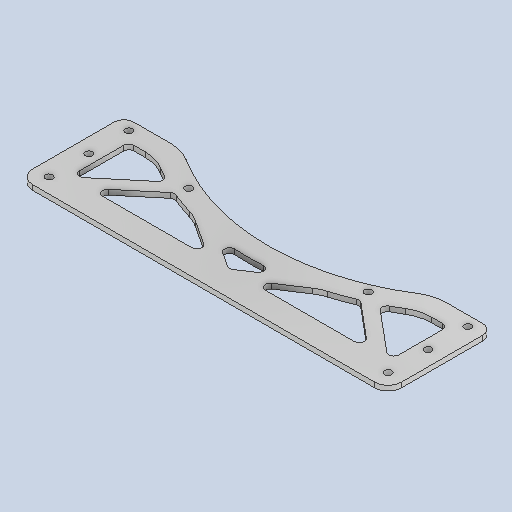
# Autodesk Inventor part: Custom Aluminum Intake
Saved by Autodesk Inventor 2025.1 (Build 291241020, 241B)
## iProperties
Created: 2024-12-30
Part Number: Custom Aluminum Intake
Material: Generic
Document SubType Name: Modeling
Designer: Juan
Density: 1 g/cm^3
Appearance: Default
Author: Juan
Autodesk Inventor part; units mm, degrees
ref_plane "YZ Plane" through (0, 0, 0) normal (1, 0, 0) x (0, 1, 0)
ref_plane "XZ Plane" through (0, 0, 0) normal (0, 1, 0) x (-1, 0, 0)
ref_plane "XY Plane" through (0, 0, 0) normal (0, 0, 1) x (1, 0, 0)
sketch "Sketch1" plane through (0, 0, 0) normal (0, 1, 0) x (-1, 0, 0)
  line L0 (0, 0) -> (-228.6, 0)
  line L1 (-228.6, 0) -> (-228.6, -82.55)
  line L2 (0, 0) -> (0, -82.55)
  line L3 (-228.6, 0) -> (-222.25, 0)
  circle A0 centre (-222.25, -6.35) radius 2.3241
  circle A1 centre (-222.25, -31.75) radius 2.3241
  line L4 (-228.6, 0) -> (-114.3, 0)
  line L5 (-114.3, 0) -> (-114.3, 9.4502)
  circle A2 centre (-222.25, -69.85) radius 2.3241
  circle A3 centre (-6.35, -6.35) radius 2.3241
  circle A4 centre (-6.35, -31.75) radius 2.3241
  circle A5 centre (-6.35, -69.85) radius 2.3241
  line L6 (-228.6, -82.55) -> (-215.9, -82.55)
  line L7 (0, -82.55) -> (-12.7, -82.55)
  line L8 (-114.3, 0) -> (-114.3, -38.1)
  arc A6 (-12.7, -82.55) -> (-215.9, -82.55) centre (-114.3, -176.4393) ccw
  line L9 (-228.6, 0) -> (-231.775, 0)
  line L10 (-231.775, 0) -> (-231.775, -82.55)
  line L11 (-231.775, -82.55) -> (-228.6, -82.55)
  line L12 (-228.6, 0) -> (-228.6, 3.175)
  line L13 (-228.6, 3.175) -> (-231.775, 3.175)
  line L14 (-231.775, 3.175) -> (-231.775, 0)
  line L15 (-228.6, 3.175) -> (0, 3.175)
  line L16 (0, 3.175) -> (0, 0)
  line L17 (0, 0) -> (3.175, 0)
  line L18 (3.175, 0) -> (3.175, 3.175)
  line L19 (3.175, 3.175) -> (0, 3.175)
  line L20 (3.175, 0) -> (3.175, -82.55)
  line L21 (3.175, -82.55) -> (0, -82.55)
  line L22 (-222.25, -69.85) -> (-222.25, -57.15)
  circle A7 centre (-222.25, -57.15) radius 2.3241
  line L23 (-6.35, -69.85) -> (-6.35, -57.15)
  circle A8 centre (-6.35, -57.15) radius 2.3241
  line L24 (-228.6, -63.5) -> (-194.1904, -63.5)
  line L25 (3.175, -63.5) -> (-34.4096, -63.5)
  line L26 (-231.775, -63.5) -> (-194.1904, -63.5)
  line L27 (-228.6, -69.85) -> (-221.3121, -69.85)
  arc A9 (-7.2879, -69.85) -> (-221.3121, -69.85) centre (-114.3, -176.4393) ccw
  line L28 (-7.2879, -69.85) -> (0, -69.85)
  line L29 (-228.6, -12.7) -> (0, -12.7)
  line L30 (-12.7, 0) -> (-12.7, -82.55)
  line L31 (-215.9, 0) -> (-215.9, -82.55)
  line L32 (-12.7, -12.7) -> (-46.8946, -41.275)
  line L33 (-12.7, -12.7) -> (-25.4, -12.7)
  line L34 (-25.4, -12.7) -> (-55.0732, -37.4966)
  line L35 (-114.3, -12.7) -> (-92.459, -26.9875)
  line L36 (-114.3, -12.7) -> (-101.6, -12.7)
  line L37 (-101.6, -12.7) -> (-73.6787, -30.965)
  line L38 (-215.9, -12.7) -> (-181.7054, -41.275)
  line L39 (-203.2, -12.7) -> (-173.5268, -37.4966)
  line L40 (-114.3, -12.7) -> (-136.141, -26.9875)
  line L41 (-127, -12.7) -> (-154.9213, -30.965)
  point P0 (-225.425, 0)
  point P1 (-215.9, -12.7)
  point P2 (-215.9, -63.5)
  point P3 (-214.5875, -63.5)
  point P4 (-14.0125, -63.5)
  point P5 (-12.7, -63.5)
  dimension "d0" = 228.6
  dimension "d1" = 82.55
  dimension "d2" = 6.35
  dimension "d4" = 4.6482
  dimension "d6" = 4.6482
  dimension "d7" = 114.3
  dimension "d9" = 4.6482
  dimension "d10" = 6.35
  dimension "d11" = 31.75
  dimension "d12" = 69.85
  dimension "d14" = 12.7
  dimension "d15" = 12.7
  dimension "d16" = 38.1
  dimension "d20" = 3.175
  dimension "d21" = 3.175
  dimension "d22" = 3.175
  dimension "d27" = 12.7
  dimension "d28" = 4.6482
  dimension "d29" = 12.7
  dimension "d30" = 4.6482
  dimension "d35" = 12.7
  dimension "d36" = 15.875
  dimension "d37" = 12.7
  dimension "d38" = 12.7
  dimension "d39" = 12.7
  dimension "d40" = 12.7
  constraints: 84 end point, 13 point on line, 11 point on circle, 10 centre point, 10 symmetric about line, 9 perpendicular, 6 parallel, 6 vertical, 4 horizontal, 3 midpoint, 2 coincident, 2 collinear, 5 other
  measures "d0" distance of L0.start L0.end
  measures "d1" distance of L0.end L1.end
  measures "d2" distance of L0.end L3.end
  measures "d4" diameter of A0
  measures "d6" diameter of A1
  measures "d7" distance of L0.end L4.end
  measures "d9" diameter of A2
  measures "d10" distance from line of A0.centre L0
  measures "d11" distance from line of L0 A1.centre
  measures "d12" vertical distance of point (-225.425, 0) L22.start
  measures "d14" distance of L1.end L6.end
  measures "d15" distance of L2.end L7.end
  measures "d16" distance of L4.end L8.end
  measures "d20" distance of L0.end L9.end
  measures "d21" distance of L0.end L12.end
  measures "d22" distance of L0.start L17.end
  measures "d27" distance of L22.start L22.end
  measures "d28" diameter of A7
  measures "d29" distance of L23.start L23.end
  measures "d30" diameter of A8
  measures "d35" radial gap between concentric circles of A6 A9
  measures "d36" distance between parallel lines of L15 L29
  measures "d37" distance between parallel lines of L2 L30
  measures "d38" distance between parallel lines of L1 L31
  measures "d39" distance of L32.start L33.end
  measures "d40" distance of L35.start L36.end
extrude "Extrusion1" add sketch "Sketch1" against normal blind 3.175 contours L2 L29 L30 L0 | L30 L29 L8 L0 | L2 L25 L30 L29 | L8 L29 L31 L0 | L32 A9 L34 L29 | L30 L25 A9 L32 | L2 L28 A5 L23 L25 | L31 L29 L1 L0 | L35 A9 L8 | L40 A9 L41 L29 | L29 L37 A9 L35 | L8 A9 L40 | L34 A9 L37 L29 | L30 A9 L25 | L25 L23 A5 A9 L30 | A9 L25 A6 L8 | L2 L7 L30 A9 A5 L28 | L31 L24 L1 L29 | L38 A9 L24 L31 | L29 L39 A9 L38 | L8 A6 L24 A9 | L41 A9 L39 L29 | A9 L30 A6 L25 | L31 A9 A2 L22 L24 | L24 A9 L31 | L24 L22 A2 L27 L1 | L24 A6 L31 A9 | L31 L6 L1 L27 A2 A9 | A7 | A8
fillet "Fillet1" radius 8.4667 4 edges at (228.6, -1.5875, -82.55) (215.9, -1.5875, -82.55) (12.7, -1.5875, -82.55) (0, -1.5875, -82.55)
extrude "Extrusion2" add sketch "Sketch1" against normal blind 3.175 contours L2 L29 L30 L0 | L17 L20 L25 L2 | L0 L5 L15 L16 | L16 L19 L18 L17 | L30 L29 L8 L0 | L2 L25 L30 L29 | L8 L29 L31 L0 | L0 L12 L15 L5 | L32 A9 L34 L29 | L30 L25 A9 L32 | L25 L20 L21 L2 | L2 L28 A5 L23 L25 | L31 L29 L1 L0 | L35 A9 L8 | L40 A9 L41 L29 | L29 L37 A9 L35 | L8 A9 L40 | L34 A9 L37 L29 | L30 A9 L25 | L25 L23 A5 A9 L30 | A9 L25 A6 L8 | L2 L7 L30 A9 A5 L28 | L12 L9 L14 L13 | L31 L24 L1 L29 | L38 A9 L24 L31 | L29 L39 A9 L38 | L8 A6 L24 A9 | L41 A9 L39 L29 | A9 L30 A6 L25 | L1 L26 L10 L9 | L31 A9 A2 L22 L24 | L24 A9 L31 | L24 L22 A2 L27 L1 | L1 L11 L10 L26 | L24 A6 L31 A9 | L31 L6 L1 L27 A2 A9 | A7 | A8
fillet "Fillet2" radius 8.4667 4 edges at (231.775, -1.5875, -82.55) (231.775, -1.5875, 3.175) (-3.175, -1.5875, 3.175) (-3.175, -1.5875, -82.55)
fillet "Fillet3" radius 12.7 2 edges at (215.9, -1.5875, -82.55) (12.7, -1.5875, -82.55)
extrude "Extrusion3" cut sketch "Sketch1" against normal blind 3.175 contours L25 L20 L21 L2 | L2 L28 A5 L23 L25 | L30 A9 L25 | L25 L23 A5 A9 L30 | L2 L7 L30 A9 A5 L28 | A9 L30 A6 L25 | L31 A9 A2 L22 L24 | L24 A9 L31 | L24 L22 A2 L27 L1 | L1 L11 L10 L26 | L24 A6 L31 A9 | L31 L6 L1 L27 A2 A9 | A7 | A8
fillet "Fillet4" radius 6.35 2 edges at (231.775, -1.5875, -63.5) (-3.175, -1.5875, -63.5)
fillet "Fillet5" radius 25.4 2 edges at (194.1904, -1.5875, -63.5) (34.4096, -1.5875, -63.5)
sketch "Sketch2" plane through (0, 0, 0) normal (0, 1, 0) x (1, 0, 0)
  arc A0 (40.2936, 59.5598) -> (26.7055, 63.5) centre (26.7055, 38.1) ccw projected
  line L0 (26.7055, 63.5) -> (3.175, 63.5) projected
  arc A1 (3.175, 63.5) -> (-3.175, 57.15) centre (3.175, 57.15) ccw projected
  line L1 (-3.175, 57.15) -> (-3.175, 5.2917) projected
  arc A2 (-3.175, 5.2917) -> (5.2917, -3.175) centre (5.2917, 5.2917) ccw projected
  line L2 (5.2917, -3.175) -> (223.3083, -3.175) projected
  arc A3 (223.3083, -3.175) -> (231.775, 5.2917) centre (223.3083, 5.2917) ccw projected
  line L3 (231.775, 5.2917) -> (231.775, 57.15) projected
  arc A4 (231.775, 57.15) -> (225.425, 63.5) centre (225.425, 57.15) ccw projected
  line L4 (225.425, 63.5) -> (201.8945, 63.5) projected
  arc A5 (201.8945, 63.5) -> (188.3064, 59.5598) centre (201.8945, 38.1) ccw projected
  arc A6 (40.2936, 59.5598) -> (188.3064, 59.5598) centre (114.3, 176.4393) ccw projected
  circle A7 centre (222.25, 57.15) radius 2.3241 projected
  circle A8 centre (6.35, 57.15) radius 2.3241 projected
  circle A9 centre (6.35, 31.75) radius 2.3241 projected
  circle A10 centre (6.35, 6.35) radius 2.3241 projected
  circle A11 centre (222.25, 6.35) radius 2.3241 projected
  circle A12 centre (222.25, 31.75) radius 2.3241 projected
  line L5 (6.35, 6.35) -> (222.25, 6.35)
  line L6 (222.25, 6.35) -> (114.3, 6.35)
  line L7 (114.3, 6.35) -> (114.3, 38.1)
  point P0 (0, 0)
  constraints: 6 end point, 1 horizontal, 1 midpoint, 1 point on circle
extrude "Extrusion4" cut sketch "Sketch1" against normal blind 3.175 contours L30 L25 A9 L32 | L35 A9 L8 | L8 A9 L40 | L34 A9 L37 L29 | L38 A9 L24 L31 | L41 A9 L39 L29
sketch "Sketch3" plane through (0, 0, 0) normal (0, 1, 0) x (1, 0, 0)
  arc A0 (40.2936, 59.5598) -> (26.7055, 63.5) centre (26.7055, 38.1) ccw projected
  line L0 (26.7055, 63.5) -> (26.7055, 50.8)
  circle A1 centre (222.25, 31.75) radius 2.3241 projected
  circle A2 centre (222.25, 6.35) radius 2.3241 projected
  circle A3 centre (6.35, 6.35) radius 2.3241 projected
  circle A4 centre (6.35, 31.75) radius 2.3241 projected
  circle A5 centre (6.35, 57.15) radius 2.3241 projected
  circle A6 centre (222.25, 57.15) radius 2.3241 projected
  arc A7 (14.0125, 63.5) -> (46.8946, 41.275) centre (114.3, 176.4393) ccw projected
  line L1 (46.8946, 41.275) -> (12.7, 12.7) projected
  line L2 (12.7, 12.7) -> (12.7, 63.5) projected
  line L3 (12.7, 63.5) -> (3.175, 63.5) projected
  arc A8 (3.175, 63.5) -> (-3.175, 57.15) centre (3.175, 57.15) ccw projected
  line L4 (-3.175, 57.15) -> (-3.175, 5.2917) projected
  arc A9 (-3.175, 5.2917) -> (5.2917, -3.175) centre (5.2917, 5.2917) ccw projected
  line L5 (5.2917, -3.175) -> (223.3083, -3.175) projected
  arc A10 (223.3083, -3.175) -> (231.775, 5.2917) centre (223.3083, 5.2917) ccw projected
  line L6 (231.775, 5.2917) -> (231.775, 57.15) projected
  arc A11 (231.775, 57.15) -> (225.425, 63.5) centre (225.425, 57.15) ccw projected
  line L7 (225.425, 63.5) -> (215.9, 63.5) projected
  line L8 (215.9, 63.5) -> (215.9, 12.7) projected
  line L9 (215.9, 12.7) -> (181.7054, 41.275) projected
  arc A12 (181.7054, 41.275) -> (214.5875, 63.5) centre (114.3, 176.4393) ccw projected
  line L10 (214.5875, 63.5) -> (201.8945, 63.5) projected
  arc A13 (201.8945, 63.5) -> (188.3064, 59.5598) centre (201.8945, 38.1) ccw projected
  arc A14 (40.2936, 59.5598) -> (188.3064, 59.5598) centre (114.3, 176.4393) ccw projected
  arc A15 (40.2936, 59.5598) -> (26.7055, 63.5) centre (26.7055, 38.1) ccw projected
  line L11 (26.7055, 63.5) -> (14.0125, 63.5) projected
  line L12 (25.4, 12.7) -> (55.0732, 37.4966) projected
  arc A16 (55.0732, 37.4966) -> (73.6787, 30.965) centre (114.3, 176.4393) ccw projected
  line L13 (73.6787, 30.965) -> (101.6, 12.7) projected
  line L14 (101.6, 12.7) -> (25.4, 12.7) projected
  line L15 (127, 12.7) -> (154.9213, 30.965) projected
  arc A17 (154.9213, 30.965) -> (173.5268, 37.4966) centre (114.3, 176.4393) ccw projected
  line L16 (173.5268, 37.4966) -> (203.2, 12.7) projected
  line L17 (203.2, 12.7) -> (127, 12.7) projected
  line L18 (114.3, 12.7) -> (92.459, 26.9875) projected
  arc A18 (92.459, 26.9875) -> (136.141, 26.9875) centre (114.3, 176.4393) ccw projected
  line L19 (136.141, 26.9875) -> (114.3, 12.7) projected
  line L20 (26.7055, 50.8) -> (12.7, 50.8)
  line L21 (26.7055, 50.8) -> (30.469, 50.8)
  line L22 (30.469, 50.8) -> (231.775, 50.8)
  line L23 (215.9, 63.5) -> (215.9, 12.7) projected
  line L24 (215.9, 50.8) -> (215.9, 63.5)
  line L25 (215.9, 63.5) -> (214.5875, 63.5)
  line L26 (198.131, 50.8) -> (214.5875, 63.5)
  line L27 (14.0125, 63.5) -> (26.7055, 63.5) projected
  line L28 (12.7, 63.5) -> (26.7055, 63.5)
  line L29 (12.7, 50.8) -> (12.7, 63.5)
  point P0 (0, 0)
  point P1 (215.9, 50.8)
  dimension "d43" = 12.7
  constraints: 18 end point, 7 point on line, 4 perpendicular, 2 point on circle, 1 horizontal, 1 vertical
  measures "d43" distance of L0.start L0.end
extrude "Extrusion5" add sketch "Sketch3" against normal blind 3.175 contours A7 L21 L0 | L0 L20 L2 L28 A7 | A12 L25 L8 L22
sketch "Sketch4" plane through (0, 0, 0) normal (0, 1, 0) x (1, 0, 0)
  circle A0 centre (6.35, 31.75) radius 2.3241 projected
  circle A1 centre (222.25, 31.75) radius 2.3241 projected
  line L0 (6.35, 31.75) -> (222.25, 31.75)
  line L1 (231.775, 57.15) -> (231.775, 5.2917) projected
  line L2 (222.25, 31.75) -> (171.45, 31.75)
  line L3 (171.45, 31.75) -> (171.45, 44.45)
  line L4 (171.45, 44.45) -> (181.1788, 36.2866)
  circle A2 centre (171.45, 44.45) radius 2.3241
  circle A3 centre (181.1788, 36.2866) radius 2.3241
  line L5 (181.1788, 36.2866) -> (155.7788, 36.2866)
  circle A4 centre (155.7788, 36.2866) radius 2.3241
  line L6 (114.3, 6.35) -> (114.3, 38.1) projected
  circle A5 centre (57.15, 44.45) radius 2.3241
  circle A6 centre (47.4212, 36.2866) radius 2.3241
  circle A7 centre (72.8212, 36.2866) radius 2.3241
  point P0 (0, 0)
  dimension "d46" = 50.8
  dimension "d47" = 12.7
  dimension "d48" = 50
  dimension "d49" = 12.7
  dimension "d50" = 4.6482
  dimension "d51" = 4.6482
  dimension "d52" = 25.4
  dimension "d53" = 4.6482
  constraints: 10 end point, 6 centre point, 3 coincident, 3 symmetric about line, 2 perpendicular, 1 horizontal, 1 point on line, 3 other
  measures "d46" distance of L0.end L2.end
  measures "d47" distance of L2.end L3.end
  measures "d48" angle of L4 L3
  measures "d49" distance of L3.end L4.end
  measures "d50" diameter of A2
  measures "d51" diameter of A3
  measures "d52" distance of L5.start L5.end
  measures "d53" diameter of A4
extrude "Extrusion6" cut sketch "Sketch4" against normal blind 3.175 contours A2 L4 L3 | L3 L4 A2 | L5 L4 A3 | A3 L4 L5 | A4 | A5 | A6 | A7
fillet "Fillet6" radius 25.4 4 edges at (73.6787, -1.5875, -30.965) (154.9213, -1.5875, -30.965) (198.131, -1.5875, -50.8) (30.469, -1.5875, -50.8)
fillet "Fillet9" radius 3.175 2 edges at (12.7, -1.5875, -50.8) (215.9, -1.5875, -50.8)
sketch "Sketch5" plane through (0, 0, 0) normal (0, 1, 0) x (1, 0, 0)
  circle A0 centre (57.15, 44.45) radius 2.3241 projected
  circle A1 centre (47.4212, 36.2866) radius 2.3241 projected
  circle A2 centre (72.8212, 36.2866) radius 2.3241 projected
  circle A3 centre (155.7788, 36.2866) radius 2.3241 projected
  circle A4 centre (171.45, 44.45) radius 2.3241 projected
  circle A5 centre (181.1788, 36.2866) radius 2.3241 projected
  arc A6 (174.2702, 36.8754) -> (172.639, 37.1216) centre (173.2522, 35.6573) ccw projected
  line L0 (173.5268, 37.4966) -> (203.2, 12.7) projected
  arc A7 (36.2266, 47.1434) -> (46.8946, 41.275) centre (114.3, 176.4393) ccw projected
  arc A8 (158.2731, 31.9428) -> (151.7632, 28.8991) centre (165.668, 7.6431) ccw projected
  arc A9 (183.8383, 42.3599) -> (183.5512, 39.7325) centre (184.5692, 40.9506) ccw projected
  line L1 (215.9, 12.7) -> (181.7054, 41.275) projected
  arc A10 (36.2266, 47.1434) -> (46.8946, 41.275) centre (114.3, 176.4393) ccw projected
  arc A11 (130.4251, 23.2484) -> (129.3974, 26.1564) centre (129.5561, 24.5769) ccw projected
  arc A12 (36.2266, 47.1434) -> (46.8946, 41.275) centre (114.3, 176.4393) ccw projected
  arc A13 (99.2026, 26.1564) -> (98.1749, 23.2484) centre (99.0439, 24.5769) ccw projected
  arc A14 (76.8368, 28.8991) -> (70.3269, 31.9428) centre (62.932, 7.6431) ccw projected
  arc A15 (36.2266, 47.1434) -> (46.8946, 41.275) centre (114.3, 176.4393) ccw projected
  line L2 (25.4, 12.7) -> (55.0732, 37.4966) projected
  arc A16 (55.961, 37.1216) -> (54.3298, 36.8754) centre (55.3478, 35.6573) ccw projected
  line L3 (46.8946, 41.275) -> (12.7, 12.7) projected
  arc A17 (45.0488, 39.7325) -> (44.7617, 42.3599) centre (44.0308, 40.9506) ccw projected
  arc A18 (36.2266, 47.1434) -> (46.8946, 41.275) centre (114.3, 176.4393) ccw projected
  point P0 (0, 0)
  point P1 (199.8426, 15.5057)
  point P2 (213.2945, 14.8773)
  point P3 (192.3734, 47.1434)
  point P4 (28.7574, 15.5057)
  point P5 (15.3055, 14.8773)
extrude "Extrusion7" add sketch "Sketch4" against normal blind 3.175 contours L5 L4 A3 | A3 L4 L5 | A4 | A6 | A7
fillet "Fillet11" radius 3.175 13 edges at (55.0732, -1.5875, -37.4966) (46.8946, -1.5875, -41.275) (12.7, -1.5875, -12.7) (25.4, -1.5875, -12.7) (101.6, -1.5875, -12.7) (92.459, -1.5875, -26.9875) (136.141, -1.5875, -26.9875) (114.3, -1.5875, -12.7) (173.5268, -1.5875, -37.4966) (127, -1.5875, -12.7) (203.2, -1.5875, -12.7) (215.9, -1.5875, -12.7) (181.7054, -1.5875, -41.275)
body "Solid1"
